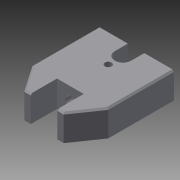
# Autodesk Inventor part: 7.2 Q6
Saved by Autodesk Inventor 2015 (Build 190159000, 159)
## iProperties
Created: 2018-02-12
Part Number: 7.2 Q6
Material: Generic
Document SubType Name: Modeling
Designer: Administrator
Density: 1 g/cm^3
Appearance: Default
Author: Administrator
Autodesk Inventor part; units mm, degrees
ref_plane "YZ Plane" through (0, 0, 0) normal (1, 0, 0) x (0, 1, 0)
ref_plane "XZ Plane" through (0, 0, 0) normal (0, 1, 0) x (-1, 0, 0)
ref_plane "XY Plane" through (0, 0, 0) normal (0, 0, 1) x (1, 0, 0)
sketch "Sketch1" plane through (0, 0, 0) normal (0, 0, 1) x (1, 0, 0)
  line L0 (0, 0) -> (88.9, 0)
  line L1 (88.9, 0) -> (88.9, 25.4)
  line L2 (88.9, 25.4) -> (0, 25.4)
  line L3 (0, 25.4) -> (0, 0)
  dimension "d0" = 25.4
  dimension "d1" = 88.9
  constraints: 8 end point, 2 parallel, 1 horizontal, 1 perpendicular
  measures "d0" distance of L2.end L0.start
  measures "d1" distance of L0.start L0.end
extrude "Extrusion1" add sketch "Sketch1" along normal blind 73.279
sketch "Sketch2" plane through (0, 25.4, 0) normal (0, 1, 0) x (1, 0, 0)
  line L0 (0, -44.4754) -> (0, -28.575)
  line L1 (0, -28.575) -> (12.7, -28.575)
  line L2 (0, -44.4754) -> (12.7, -44.4754)
  arc A0 (12.7, -44.4754) -> (12.7, -28.575) centre (12.7, -36.5252) ccw
  line L3 (88.9, 0) -> (0, 0) projected
  line L4 (0, 0) -> (0, -73.279) projected
  dimension "d5" = 36.5252
  dimension "d6" = 7.9502
  dimension "d7" = 12.7
  dimension "d8" = 0
  dimension "d9" = 12.7
  dimension "d10" = 12.7
  constraints: 6 end point, 2 point on circle, 1 centre point, 1 horizontal, 1 perpendicular
  measures "d5" vertical distance of A0.centre L3.end
  measures "d6" radius of A0
  measures "d7" distance from line of L4 A0.centre
  measures "d8" distance between parallel lines of L4 L0
  measures "d9" distance of L0.end L1.end
  measures "d10" distance of L0.start L2.end
extrude "Extrusion2" cut sketch "Sketch2" against normal blind 73.279
sketch "Sketch3" plane through (0, 25.4, 0) normal (0, 1, 0) x (1, 0, 0)
  line L0 (0, -73.279) -> (88.9, -73.279) projected
  line L1 (63.5, -73.279) -> (88.9, -55.753)
  line L2 (88.9, 0) -> (88.9, -73.279) projected
  line L3 (88.9, -73.279) -> (63.5, -73.279)
  line L4 (88.9, -73.279) -> (88.9, -55.753)
  line L5 (63.5, 0) -> (88.9, 0)
  line L6 (88.9, 0) -> (0, 0) projected
  line L7 (88.9, -17.526) -> (63.5, 0)
  line L8 (88.9, -17.526) -> (88.9, 0)
  line L9 (0, -44.4754) -> (0, -73.279) projected
  line L10 (0, 0) -> (0, -28.575) projected
  dimension "d13" = 17.526
  dimension "d14" = 17.526
  dimension "d15" = 63.5
  dimension "d16" = 63.5
  constraints: 12 end point, 3 point on line, 2 collinear, 1 vertical
  measures "d13" distance from line of L1.end L0
  measures "d14" distance of L2.start L7.start
  measures "d15" distance from line of L9 L1.start
  measures "d16" distance from line of L10 L5.start
extrude "Extrusion3" cut sketch "Sketch3" against normal blind 73.279
sketch "Sketch4" plane through (88.9, 0, 55.753) normal (1, 0, 0) x (0, 0, -1)
  line L0 (0, 25.4) -> (0, 0) projected
  line L1 (55.753, 25.4) -> (27.178, 25.4) projected
  line L2 (6.2992, 0) -> (32.0802, 0)
  line L3 (32.0802, 0) -> (32.0802, 25.4)
  line L4 (32.0802, 25.4) -> (6.2992, 25.4)
  line L5 (6.2992, 25.4) -> (6.2992, 0)
  line L6 (-17.526, 0) -> (-17.526, 25.4) projected
  point P0 (55.753, 0)
  dimension "d19" = 25.781
  dimension "d20" = 23.8252
  constraints: 8 end point, 2 parallel, 1 horizontal, 1 perpendicular, 1 point on line
  measures "d19" distance of L2.start L2.end
  measures "d20" distance between parallel lines of L6 L5
extrude "Extrusion4" cut sketch "Sketch4" against normal blind 25.4
chamfer "Chamfer1" distance 1.524 angle 45 6 edges at (31.75, 25.4, 73.279) (76.2, 25.4, 64.516) (88.9, 25.4, 52.6034) (88.9, 25.4, 20.5994) (76.2, 25.4, 8.763) (31.75, 25.4, 0)
sketch "Sketch5" plane through (0, 25.4, 28.575) normal (0, 1, 0) x (1, 0, 0)
  line L0 (0, 27.051) -> (0, 0) projected
  line L1 (63.5, 28.575) -> (0, 28.575) projected
  point P0 (26.9748, -7.9502)
  dimension "d26" = 26.9748
  dimension "d27" = 36.5252
  measures "d26" distance from line of L0 point (26.975, -7.95)
  measures "d27" distance from line of L1 point (26.975, -7.95)
hole "Hole1" at (26.9748, 25.4, 36.5252) direction (0, -1, 0) diameter 6.477 depth 14.2748 tip angle 118
sketch "Sketch6" plane through (63.5, 0, 55.753) normal (1, 0, 0) x (0, 0, -1)
  line L0 (6.2992, 25.4) -> (32.0802, 25.4) projected
  line L1 (6.2992, 0) -> (6.2992, 23.876) projected
  point P0 (55.753, 0)
  point P1 (19.1897, 12.7)
  dimension "d35" = 12.7
  dimension "d36" = 12.8905
  measures "d35" distance from line of point (19.19, 12.7) L0
  measures "d36" distance from line of L1 point (19.19, 12.7)
hole "Hole2" at (63.5, 12.7, 36.5633) direction (-1, 0, 0) diameter 9.525 depth 19.05 tip angle 118
body "Solid1"
